Autodesk Inventor part; units mm, degrees
(part 12 of 13)
  line L4314 (13.4922, 7.2115) -> (13.6786, 7.3979)
  arc A4310 (13.6786, 7.3979) -> (13.5708, 7.5057) centre (13.6247, 7.4518) ccw
  line L4315 (13.5708, 7.5057) -> (13.3844, 7.3193)
  arc A4311 (13.3844, 7.3193) -> (13.4922, 7.2115) centre (13.4383, 7.2654) ccw
  line L4316 (13.7009, 7.4518) -> (13.7009, 7.8246)
  arc A4312 (13.7009, 7.8246) -> (13.5485, 7.8246) centre (13.6247, 7.8246) ccw
  line L4317 (13.5485, 7.8246) -> (13.5485, 7.4518)
  arc A4313 (13.5485, 7.4518) -> (13.7009, 7.4518) centre (13.6247, 7.4518) ccw
  line L4318 (13.6786, 7.8785) -> (13.4922, 8.065)
  arc A4314 (13.4922, 8.065) -> (13.3844, 7.9572) centre (13.4383, 8.0111) ccw
  line L4319 (13.3844, 7.9572) -> (13.5708, 7.7707)
  arc A4315 (13.5708, 7.7707) -> (13.6786, 7.8785) centre (13.6247, 7.8246) ccw
  line L4320 (13.4383, 8.0873) -> (12.6926, 8.0873)
  arc A4316 (12.6926, 8.0873) -> (12.6926, 7.9349) centre (12.6926, 8.0111) ccw
  line L4321 (12.6926, 7.9349) -> (13.4383, 7.9349)
  line L4322 (12.6387, 8.065) -> (12.4523, 7.8785)
  arc A4317 (12.4523, 7.8785) -> (12.5601, 7.7707) centre (12.5062, 7.8246) ccw
  line L4323 (12.5601, 7.7707) -> (12.7465, 7.9572)
  arc A4318 (12.7465, 7.9572) -> (12.6387, 8.065) centre (12.6926, 8.0111) ccw
  line L4324 (12.43, 7.8246) -> (12.43, 7.4518)
  arc A4319 (12.43, 7.4518) -> (12.5824, 7.4518) centre (12.5062, 7.4518) ccw
  line L4325 (12.5824, 7.4518) -> (12.5824, 7.8246)
  arc A4320 (12.5824, 7.8246) -> (12.43, 7.8246) centre (12.5062, 7.8246) ccw
  line L4326 (12.4523, 7.3979) -> (12.6387, 7.2115)
  arc A4321 (12.6387, 7.2115) -> (12.7465, 7.3193) centre (12.6926, 7.2654) ccw
  line L4327 (12.7465, 7.3193) -> (12.5601, 7.5057)
  arc A4322 (12.5601, 7.5057) -> (12.4523, 7.3979) centre (12.5062, 7.4518) ccw
  line L4328 (12.7465, 7.2115) -> (13.4922, 7.9572)
  arc A4323 (13.4922, 7.9572) -> (13.3844, 8.065) centre (13.4383, 8.0111) ccw
  line L4329 (13.3844, 8.065) -> (12.6387, 7.3193)
  arc A4324 (12.6387, 7.3193) -> (12.7465, 7.2115) centre (12.6926, 7.2654) ccw
  line L4330 (13.3058, 8.3808) -> (13.6786, 8.7536)
  arc A4325 (13.6786, 8.7536) -> (13.5708, 8.8614) centre (13.6247, 8.8075) ccw
  line L4331 (13.5708, 8.8614) -> (13.198, 8.4886)
  arc A4326 (13.198, 8.4886) -> (13.3058, 8.3808) centre (13.2519, 8.4347) ccw
  line L4332 (13.6247, 8.8837) -> (12.5062, 8.8837)
  arc A4327 (12.5062, 8.8837) -> (12.5062, 8.7313) centre (12.5062, 8.8075) ccw
  line L4333 (12.5062, 8.7313) -> (13.6247, 8.7313)
  arc A4328 (13.6247, 8.7313) -> (13.6247, 8.8837) centre (13.6247, 8.8075) ccw
  line L4334 (12.5824, 8.4347) -> (12.5824, 9.1804)
  arc A4329 (12.5824, 9.1804) -> (12.43, 9.1804) centre (12.5062, 9.1804) ccw
  line L4335 (12.43, 9.1804) -> (12.43, 8.4347)
  arc A4330 (12.43, 8.4347) -> (12.5824, 8.4347) centre (12.5062, 8.4347) ccw
  line L4336 (13.4922, 9.5501) -> (13.6786, 9.7365)
  arc A4331 (13.6786, 9.7365) -> (13.5708, 9.8443) centre (13.6247, 9.7904) ccw
  line L4337 (13.5708, 9.8443) -> (13.3844, 9.6579)
  arc A4332 (13.3844, 9.6579) -> (13.4922, 9.5501) centre (13.4383, 9.604) ccw
  line L4338 (13.7009, 9.7904) -> (13.7009, 10.1632)
  arc A4333 (13.7009, 10.1632) -> (13.5485, 10.1632) centre (13.6247, 10.1632) ccw
  line L4339 (13.5485, 10.1632) -> (13.5485, 9.7904)
  arc A4334 (13.5485, 9.7904) -> (13.7009, 9.7904) centre (13.6247, 9.7904) ccw
  line L4340 (13.6786, 10.2171) -> (13.4922, 10.4036)
  arc A4335 (13.4922, 10.4036) -> (13.3844, 10.2958) centre (13.4383, 10.3497) ccw
  line L4341 (13.3844, 10.2958) -> (13.5708, 10.1093)
  arc A4336 (13.5708, 10.1093) -> (13.6786, 10.2171) centre (13.6247, 10.1632) ccw
  line L4342 (13.4383, 10.4259) -> (13.2519, 10.4259)
  arc A4337 (13.2519, 10.4259) -> (13.2519, 10.2735) centre (13.2519, 10.3497) ccw
  line L4343 (13.2519, 10.2735) -> (13.4383, 10.2735)
  arc A4338 (13.4383, 10.2735) -> (13.4383, 10.4259) centre (13.4383, 10.3497) ccw
  line L4344 (13.198, 10.4036) -> (13.0115, 10.2171)
  arc A4339 (13.0115, 10.2171) -> (13.1193, 10.1093) centre (13.0654, 10.1632) ccw
  line L4345 (13.1193, 10.1093) -> (13.3058, 10.2958)
  arc A4340 (13.3058, 10.2958) -> (13.198, 10.4036) centre (13.2519, 10.3497) ccw
  line L4346 (13.1193, 10.2171) -> (12.9329, 10.4036)
  arc A4341 (12.9329, 10.4036) -> (12.8251, 10.2958) centre (12.879, 10.3497) ccw
  line L4347 (12.8251, 10.2958) -> (13.0115, 10.1093)
  arc A4342 (13.0115, 10.1093) -> (13.1193, 10.2171) centre (13.0654, 10.1632) ccw
  line L4348 (12.879, 10.4259) -> (12.6926, 10.4259)
  arc A4343 (12.6926, 10.4259) -> (12.6926, 10.2735) centre (12.6926, 10.3497) ccw
  line L4349 (12.6926, 10.2735) -> (12.879, 10.2735)
  arc A4344 (12.879, 10.2735) -> (12.879, 10.4259) centre (12.879, 10.3497) ccw
  line L4350 (12.6387, 10.4036) -> (12.4523, 10.2171)
  arc A4345 (12.4523, 10.2171) -> (12.5601, 10.1093) centre (12.5062, 10.1632) ccw
  line L4351 (12.5601, 10.1093) -> (12.7465, 10.2958)
  arc A4346 (12.7465, 10.2958) -> (12.6387, 10.4036) centre (12.6926, 10.3497) ccw
  line L4352 (12.43, 10.1632) -> (12.43, 9.7904)
  arc A4347 (12.43, 9.7904) -> (12.5824, 9.7904) centre (12.5062, 9.7904) ccw
  line L4353 (12.5824, 9.7904) -> (12.5824, 10.1632)
  arc A4348 (12.5824, 10.1632) -> (12.43, 10.1632) centre (12.5062, 10.1632) ccw
  line L4354 (12.4523, 9.7365) -> (12.6387, 9.5501)
  arc A4349 (12.6387, 9.5501) -> (12.7465, 9.6579) centre (12.6926, 9.604) ccw
  line L4355 (12.7465, 9.6579) -> (12.5601, 9.8443)
  arc A4350 (12.5601, 9.8443) -> (12.4523, 9.7365) centre (12.5062, 9.7904) ccw
  line L4356 (12.6926, 9.5278) -> (12.879, 9.5278)
  arc A4351 (12.879, 9.5278) -> (12.879, 9.6802) centre (12.879, 9.604) ccw
  line L4357 (12.879, 9.6802) -> (12.6926, 9.6802)
  arc A4352 (12.6926, 9.6802) -> (12.6926, 9.5278) centre (12.6926, 9.604) ccw
  line L4358 (12.9329, 9.5501) -> (13.1193, 9.7365)
  arc A4353 (13.1193, 9.7365) -> (13.0115, 9.8443) centre (13.0654, 9.7904) ccw
  line L4359 (13.0115, 9.8443) -> (12.8251, 9.6579)
  arc A4354 (12.8251, 9.6579) -> (12.9329, 9.5501) centre (12.879, 9.604) ccw
  line L4360 (13.0115, 9.7365) -> (13.198, 9.5501)
  arc A4355 (13.198, 9.5501) -> (13.3058, 9.6579) centre (13.2519, 9.604) ccw
  line L4361 (13.3058, 9.6579) -> (13.1193, 9.8443)
  arc A4356 (13.1193, 9.8443) -> (13.0115, 9.7365) centre (13.0654, 9.7904) ccw
  line L4362 (13.2519, 9.5278) -> (13.4383, 9.5278)
  arc A4357 (13.4383, 9.5278) -> (13.4383, 9.6802) centre (13.4383, 9.604) ccw
  line L4363 (13.4383, 9.6802) -> (13.2519, 9.6802)
  arc A4358 (13.2519, 9.6802) -> (13.2519, 9.5278) centre (13.2519, 9.604) ccw
  line L4364 (13.1416, 9.7904) -> (13.1416, 10.1632)
  arc A4359 (13.1416, 10.1632) -> (12.9892, 10.1632) centre (13.0654, 10.1632) ccw
  line L4365 (12.9892, 10.1632) -> (12.9892, 9.7904)
  arc A4360 (12.9892, 9.7904) -> (13.1416, 9.7904) centre (13.0654, 9.7904) ccw
  line L4366 (12.5062, 11.8664) -> (13.6247, 11.8664)
  arc A4361 (13.6247, 11.8664) -> (13.6247, 12.0188) centre (13.6247, 11.9426) ccw
  line L4367 (13.6247, 12.0188) -> (12.5062, 12.0188)
  arc A4362 (12.5062, 12.0188) -> (12.5062, 11.8664) centre (12.5062, 11.9426) ccw
  line L4368 (13.7009, 11.9426) -> (13.7009, 12.5018)
  arc A4363 (13.7009, 12.5018) -> (13.5485, 12.5018) centre (13.6247, 12.5018) ccw
  line L4369 (13.5485, 12.5018) -> (13.5485, 11.9426)
  arc A4364 (13.5485, 11.9426) -> (13.7009, 11.9426) centre (13.6247, 11.9426) ccw
  line L4370 (13.6786, 12.5557) -> (13.4922, 12.7422)
  arc A4365 (13.4922, 12.7422) -> (13.3844, 12.6344) centre (13.4383, 12.6883) ccw
  line L4371 (13.3844, 12.6344) -> (13.5708, 12.4479)
  arc A4366 (13.5708, 12.4479) -> (13.6786, 12.5557) centre (13.6247, 12.5018) ccw
  line L4372 (13.4383, 12.7645) -> (13.0654, 12.7645)
  arc A4367 (13.0654, 12.7645) -> (13.0654, 12.6121) centre (13.0654, 12.6883) ccw
  line L4373 (13.0654, 12.6121) -> (13.4383, 12.6121)
  arc A4368 (13.4383, 12.6121) -> (13.4383, 12.7645) centre (13.4383, 12.6883) ccw
  line L4374 (13.0115, 12.7422) -> (12.8251, 12.5557)
  arc A4369 (12.8251, 12.5557) -> (12.9329, 12.4479) centre (12.879, 12.5018) ccw
  line L4375 (12.9329, 12.4479) -> (13.1193, 12.6344)
  arc A4370 (13.1193, 12.6344) -> (13.0115, 12.7422) centre (13.0654, 12.6883) ccw
  line L4376 (12.8028, 12.5018) -> (12.8028, 11.9426)
  arc A4371 (12.8028, 11.9426) -> (12.9552, 11.9426) centre (12.879, 11.9426) ccw
  line L4377 (12.9552, 11.9426) -> (12.9552, 12.5018)
  arc A4372 (12.9552, 12.5018) -> (12.8028, 12.5018) centre (12.879, 12.5018) ccw
  line L4378 (12.9329, 12.3693) -> (12.5601, 12.7422)
  arc A4373 (12.5601, 12.7422) -> (12.4523, 12.6344) centre (12.5062, 12.6883) ccw
  line L4379 (12.4523, 12.6344) -> (12.8251, 12.2615)
  arc A4374 (12.8251, 12.2615) -> (12.9329, 12.3693) centre (12.879, 12.3154) ccw
  line L4380 (12.5062, 14.205) -> (13.6247, 14.205)
  arc A4375 (13.6247, 14.205) -> (13.6247, 14.3574) centre (13.6247, 14.2812) ccw
  line L4381 (13.6247, 14.3574) -> (12.5062, 14.3574)
  arc A4376 (12.5062, 14.3574) -> (12.5062, 14.205) centre (12.5062, 14.2812) ccw
  line L4382 (13.7009, 14.2812) -> (13.7009, 14.8404)
  arc A4377 (13.7009, 14.8404) -> (13.5485, 14.8404) centre (13.6247, 14.8404) ccw
  line L4383 (13.5485, 14.8404) -> (13.5485, 14.2812)
  arc A4378 (13.5485, 14.2812) -> (13.7009, 14.2812) centre (13.6247, 14.2812) ccw
  line L4384 (13.6786, 14.8943) -> (13.4922, 15.0808)
  arc A4379 (13.4922, 15.0808) -> (13.3844, 14.973) centre (13.4383, 15.0269) ccw
  line L4385 (13.3844, 14.973) -> (13.5708, 14.7865)
  arc A4380 (13.5708, 14.7865) -> (13.6786, 14.8943) centre (13.6247, 14.8404) ccw
  line L4386 (13.4383, 15.1031) -> (13.0654, 15.1031)
  arc A4381 (13.0654, 15.1031) -> (13.0654, 14.9507) centre (13.0654, 15.0269) ccw
  line L4387 (13.0654, 14.9507) -> (13.4383, 14.9507)
  arc A4382 (13.4383, 14.9507) -> (13.4383, 15.1031) centre (13.4383, 15.0269) ccw
  line L4388 (13.0115, 15.0808) -> (12.8251, 14.8943)
  arc A4383 (12.8251, 14.8943) -> (12.9329, 14.7865) centre (12.879, 14.8404) ccw
  line L4389 (12.9329, 14.7865) -> (13.1193, 14.973)
  arc A4384 (13.1193, 14.973) -> (13.0115, 15.0808) centre (13.0654, 15.0269) ccw
  line L4390 (12.8028, 14.8404) -> (12.8028, 14.2812)
  arc A4385 (12.8028, 14.2812) -> (12.9552, 14.2812) centre (12.879, 14.2812) ccw
  line L4391 (12.9552, 14.2812) -> (12.9552, 14.8404)
  arc A4386 (12.9552, 14.8404) -> (12.8028, 14.8404) centre (12.879, 14.8404) ccw
  line L4392 (12.9329, 14.7079) -> (12.5601, 15.0808)
  arc A4387 (12.5601, 15.0808) -> (12.4523, 14.973) centre (12.5062, 15.0269) ccw
  line L4393 (12.4523, 14.973) -> (12.8251, 14.6001)
  arc A4388 (12.8251, 14.6001) -> (12.9329, 14.7079) centre (12.879, 14.654) ccw
  line L4394 (12.5062, 15.3743) -> (13.2519, 15.3743)
  arc A4389 (13.2519, 15.3743) -> (13.2519, 15.5267) centre (13.2519, 15.4505) ccw
  line L4395 (13.2519, 15.5267) -> (12.5062, 15.5267)
  arc A4390 (12.5062, 15.5267) -> (12.5062, 15.3743) centre (12.5062, 15.4505) ccw
  line L4396 (13.3058, 15.3966) -> (13.6786, 15.7694)
  arc A4391 (13.6786, 15.7694) -> (13.5708, 15.8772) centre (13.6247, 15.8233) ccw
  line L4397 (13.5708, 15.8772) -> (13.198, 15.5044)
  arc A4392 (13.198, 15.5044) -> (13.3058, 15.3966) centre (13.2519, 15.4505) ccw
  line L4398 (13.6786, 15.8772) -> (13.3058, 16.2501)
  arc A4393 (13.3058, 16.2501) -> (13.198, 16.1423) centre (13.2519, 16.1962) ccw
  line L4399 (13.198, 16.1423) -> (13.5708, 15.7694)
  arc A4394 (13.5708, 15.7694) -> (13.6786, 15.8772) centre (13.6247, 15.8233) ccw
  line L4400 (13.2519, 16.2724) -> (12.5062, 16.2724)
  arc A4395 (12.5062, 16.2724) -> (12.5062, 16.12) centre (12.5062, 16.1962) ccw
  line L4401 (12.5062, 16.12) -> (13.2519, 16.12)
  arc A4396 (13.2519, 16.12) -> (13.2519, 16.2724) centre (13.2519, 16.1962) ccw
  line L4402 (13.1416, 15.4505) -> (13.1416, 16.1962)
  arc A4397 (13.1416, 16.1962) -> (12.9892, 16.1962) centre (13.0654, 16.1962) ccw
  line L4403 (12.9892, 16.1962) -> (12.9892, 15.4505)
  arc A4398 (12.9892, 15.4505) -> (13.1416, 15.4505) centre (13.0654, 15.4505) ccw
  line L4404 (13.6247, 16.696) -> (12.5062, 16.696)
  arc A4399 (12.5062, 16.696) -> (12.5062, 16.5436) centre (12.5062, 16.6198) ccw
  line L4405 (12.5062, 16.5436) -> (13.6247, 16.5436)
  arc A4400 (13.6247, 16.5436) -> (13.6247, 16.696) centre (13.6247, 16.6198) ccw
  line L4406 (12.5824, 16.6198) -> (12.5824, 17.179)
  arc A4401 (12.5824, 17.179) -> (12.43, 17.179) centre (12.5062, 17.179) ccw
  line L4407 (12.43, 17.179) -> (12.43, 16.6198)
  arc A4402 (12.43, 16.6198) -> (12.5824, 16.6198) centre (12.5062, 16.6198) ccw
  line L4408 (12.5601, 17.1251) -> (12.7465, 17.3116)
  arc A4403 (12.7465, 17.3116) -> (12.6387, 17.4194) centre (12.6926, 17.3655) ccw
  line L4409 (12.6387, 17.4194) -> (12.4523, 17.2329)
  arc A4404 (12.4523, 17.2329) -> (12.5601, 17.1251) centre (12.5062, 17.179) ccw
  line L4410 (12.6926, 17.2893) -> (13.4383, 17.2893)
  arc A4405 (13.4383, 17.2893) -> (13.4383, 17.4417) centre (13.4383, 17.3655) ccw
  line L4411 (13.4383, 17.4417) -> (12.6926, 17.4417)
  arc A4406 (12.6926, 17.4417) -> (12.6926, 17.2893) centre (12.6926, 17.3655) ccw
  line L4412 (13.3844, 17.3116) -> (13.5708, 17.1251)
  arc A4407 (13.5708, 17.1251) -> (13.6786, 17.2329) centre (13.6247, 17.179) ccw
  line L4413 (13.6786, 17.2329) -> (13.4922, 17.4194)
  arc A4408 (13.4922, 17.4194) -> (13.3844, 17.3116) centre (13.4383, 17.3655) ccw
  line L4414 (13.5485, 17.179) -> (13.5485, 16.6198)
  arc A4409 (13.5485, 16.6198) -> (13.7009, 16.6198) centre (13.6247, 16.6198) ccw
  line L4415 (13.7009, 16.6198) -> (13.7009, 17.179)
  arc A4410 (13.7009, 17.179) -> (13.5485, 17.179) centre (13.6247, 17.179) ccw
  line L4416 (13.5485, 18.5348) -> (13.5485, 17.7891)
  arc A4411 (13.5485, 17.7891) -> (13.7009, 17.7891) centre (13.6247, 17.7891) ccw
  line L4417 (13.7009, 17.7891) -> (13.7009, 18.5348)
  arc A4412 (13.7009, 18.5348) -> (13.5485, 18.5348) centre (13.6247, 18.5348) ccw
  line L4418 (13.6247, 17.8653) -> (12.5062, 17.8653)
  arc A4413 (12.5062, 17.8653) -> (12.5062, 17.7129) centre (12.5062, 17.7891) ccw
  line L4419 (12.5062, 17.7129) -> (13.6247, 17.7129)
  arc A4414 (13.6247, 17.7129) -> (13.6247, 17.8653) centre (13.6247, 17.7891) ccw
  line L4420 (12.5824, 17.7891) -> (12.5824, 18.5348)
  arc A4415 (12.5824, 18.5348) -> (12.43, 18.5348) centre (12.5062, 18.5348) ccw
  line L4421 (12.43, 18.5348) -> (12.43, 17.7891)
  arc A4416 (12.43, 17.7891) -> (12.5824, 17.7891) centre (12.5062, 17.7891) ccw
  line L4422 (13.1416, 17.7891) -> (13.1416, 18.1619)
  arc A4417 (13.1416, 18.1619) -> (12.9892, 18.1619) centre (13.0654, 18.1619) ccw
  line L4423 (12.9892, 18.1619) -> (12.9892, 17.7891)
  arc A4418 (12.9892, 17.7891) -> (13.1416, 17.7891) centre (13.0654, 17.7891) ccw
  line L4424 (12.5062, 18.8822) -> (13.6247, 18.8822)
  arc A4419 (13.6247, 18.8822) -> (13.6247, 19.0346) centre (13.6247, 18.9584) ccw
  line L4425 (13.6247, 19.0346) -> (12.5062, 19.0346)
  arc A4420 (12.5062, 19.0346) -> (12.5062, 18.8822) centre (12.5062, 18.9584) ccw
  line L4426 (13.6786, 19.0123) -> (13.3058, 19.3851)
  arc A4421 (13.3058, 19.3851) -> (13.198, 19.2773) centre (13.2519, 19.3312) ccw
  line L4427 (13.198, 19.2773) -> (13.5708, 18.9045)
  arc A4422 (13.5708, 18.9045) -> (13.6786, 19.0123) centre (13.6247, 18.9584) ccw
  line L4428 (13.3058, 19.2773) -> (13.6786, 19.6502)
  arc A4423 (13.6786, 19.6502) -> (13.5708, 19.758) centre (13.6247, 19.7041) ccw
  line L4429 (13.5708, 19.758) -> (13.198, 19.3851)
  arc A4424 (13.198, 19.3851) -> (13.3058, 19.2773) centre (13.2519, 19.3312) ccw
  line L4430 (13.6247, 19.7803) -> (12.5062, 19.7803)
  arc A4425 (12.5062, 19.7803) -> (12.5062, 19.6279) centre (12.5062, 19.7041) ccw
  line L4431 (12.5062, 19.6279) -> (13.6247, 19.6279)
  arc A4426 (13.6247, 19.6279) -> (13.6247, 19.7803) centre (13.6247, 19.7041) ccw
  line L4432 (12.5062, 20.0515) -> (13.2519, 20.0515)
  arc A4427 (13.2519, 20.0515) -> (13.2519, 20.2039) centre (13.2519, 20.1277) ccw
  line L4433 (13.2519, 20.2039) -> (12.5062, 20.2039)
  arc A4428 (12.5062, 20.2039) -> (12.5062, 20.0515) centre (12.5062, 20.1277) ccw
  line L4434 (13.3058, 20.0738) -> (13.6786, 20.4466)
  arc A4429 (13.6786, 20.4466) -> (13.5708, 20.5544) centre (13.6247, 20.5005) ccw
  line L4435 (13.5708, 20.5544) -> (13.198, 20.1816)
  arc A4430 (13.198, 20.1816) -> (13.3058, 20.0738) centre (13.2519, 20.1277) ccw
  line L4436 (13.6786, 20.5544) -> (13.3058, 20.9273)
  arc A4431 (13.3058, 20.9273) -> (13.198, 20.8195) centre (13.2519, 20.8734) ccw
  line L4437 (13.198, 20.8195) -> (13.5708, 20.4466)
  arc A4432 (13.5708, 20.4466) -> (13.6786, 20.5544) centre (13.6247, 20.5005) ccw
  line L4438 (13.2519, 20.9496) -> (12.5062, 20.9496)
  arc A4433 (12.5062, 20.9496) -> (12.5062, 20.7972) centre (12.5062, 20.8734) ccw
  line L4439 (12.5062, 20.7972) -> (13.2519, 20.7972)
  arc A4434 (13.2519, 20.7972) -> (13.2519, 20.9496) centre (13.2519, 20.8734) ccw
  line L4440 (13.1416, 20.1277) -> (13.1416, 20.8734)
  arc A4435 (13.1416, 20.8734) -> (12.9892, 20.8734) centre (13.0654, 20.8734) ccw
  line L4441 (12.9892, 20.8734) -> (12.9892, 20.1277)
  arc A4436 (12.9892, 20.1277) -> (13.1416, 20.1277) centre (13.0654, 20.1277) ccw
  line L4442 (13.3844, 21.9888) -> (13.5708, 21.8023)
  arc A4437 (13.5708, 21.8023) -> (13.6786, 21.9101) centre (13.6247, 21.8562) ccw
  line L4443 (13.6786, 21.9101) -> (13.4922, 22.0966)
  arc A4438 (13.4922, 22.0966) -> (13.3844, 21.9888) centre (13.4383, 22.0427) ccw
  line L4444 (13.5485, 21.8562) -> (13.5485, 21.4834)
  arc A4439 (13.5485, 21.4834) -> (13.7009, 21.4834) centre (13.6247, 21.4834) ccw
  line L4445 (13.7009, 21.4834) -> (13.7009, 21.8562)
  arc A4440 (13.7009, 21.8562) -> (13.5485, 21.8562) centre (13.6247, 21.8562) ccw
  line L4446 (13.5708, 21.5373) -> (13.3844, 21.3509)
  arc A4441 (13.3844, 21.3509) -> (13.4922, 21.2431) centre (13.4383, 21.297) ccw
  line L4447 (13.4922, 21.2431) -> (13.6786, 21.4295)
  arc A4442 (13.6786, 21.4295) -> (13.5708, 21.5373) centre (13.6247, 21.4834) ccw
  line L4448 (13.4383, 21.3732) -> (12.6926, 21.3732)
  arc A4443 (12.6926, 21.3732) -> (12.6926, 21.2208) centre (12.6926, 21.297) ccw
  line L4449 (12.6926, 21.2208) -> (13.4383, 21.2208)
  arc A4444 (13.4383, 21.2208) -> (13.4383, 21.3732) centre (13.4383, 21.297) ccw
  line L4450 (12.7465, 21.3509) -> (12.5601, 21.5373)
  arc A4445 (12.5601, 21.5373) -> (12.4523, 21.4295) centre (12.5062, 21.4834) ccw
  line L4451 (12.4523, 21.4295) -> (12.6387, 21.2431)
  arc A4446 (12.6387, 21.2431) -> (12.7465, 21.3509) centre (12.6926, 21.297) ccw
  line L4452 (12.5824, 21.4834) -> (12.5824, 21.8562)
  arc A4447 (12.5824, 21.8562) -> (12.43, 21.8562) centre (12.5062, 21.8562) ccw
  line L4453 (12.43, 21.8562) -> (12.43, 21.4834)
  arc A4448 (12.43, 21.4834) -> (12.5824, 21.4834) centre (12.5062, 21.4834) ccw
  line L4454 (12.5601, 21.8023) -> (12.7465, 21.9888)
  arc A4449 (12.7465, 21.9888) -> (12.6387, 22.0966) centre (12.6926, 22.0427) ccw
  line L4455 (12.6387, 22.0966) -> (12.4523, 21.9101)
  arc A4450 (12.4523, 21.9101) -> (12.5601, 21.8023) centre (12.5062, 21.8562) ccw
  line L4456 (12.5062, 22.3901) -> (13.6247, 22.3901)
  arc A4451 (13.6247, 22.3901) -> (13.6247, 22.5425) centre (13.6247, 22.4663) ccw
  line L4457 (13.6247, 22.5425) -> (12.5062, 22.5425)
  arc A4452 (12.5062, 22.5425) -> (12.5062, 22.3901) centre (12.5062, 22.4663) ccw
  line L4458 (13.1416, 22.4663) -> (13.1416, 23.212)
  arc A4453 (13.1416, 23.212) -> (12.9892, 23.212) centre (13.0654, 23.212) ccw
  line L4459 (12.9892, 23.212) -> (12.9892, 22.4663)
  arc A4454 (12.9892, 22.4663) -> (13.1416, 22.4663) centre (13.0654, 22.4663) ccw
  line L4460 (13.6247, 23.2882) -> (12.5062, 23.2882)
  arc A4455 (12.5062, 23.2882) -> (12.5062, 23.1358) centre (12.5062, 23.212) ccw
  line L4461 (12.5062, 23.1358) -> (13.6247, 23.1358)
  arc A4456 (13.6247, 23.1358) -> (13.6247, 23.2882) centre (13.6247, 23.212) ccw
  line L4462 (13.5485, 24.3813) -> (13.5485, 23.6356)
  arc A4457 (13.5485, 23.6356) -> (13.7009, 23.6356) centre (13.6247, 23.6356) ccw
  line L4463 (13.7009, 23.6356) -> (13.7009, 24.3813)
  arc A4458 (13.7009, 24.3813) -> (13.5485, 24.3813) centre (13.6247, 24.3813) ccw
  line L4464 (13.6247, 23.7118) -> (12.5062, 23.7118)
  arc A4459 (12.5062, 23.7118) -> (12.5062, 23.5594) centre (12.5062, 23.6356) ccw
  line L4465 (12.5062, 23.5594) -> (13.6247, 23.5594)
  arc A4460 (13.6247, 23.5594) -> (13.6247, 23.7118) centre (13.6247, 23.6356) ccw
  line L4466 (12.5824, 23.6356) -> (12.5824, 24.3813)
  arc A4461 (12.5824, 24.3813) -> (12.43, 24.3813) centre (12.5062, 24.3813) ccw
  line L4467 (12.43, 24.3813) -> (12.43, 23.6356)
  arc A4462 (12.43, 23.6356) -> (12.5824, 23.6356) centre (12.5062, 23.6356) ccw
  line L4468 (13.1416, 23.6356) -> (13.1416, 24.0084)
  arc A4463 (13.1416, 24.0084) -> (12.9892, 24.0084) centre (13.0654, 24.0084) ccw
  line L4469 (12.9892, 24.0084) -> (12.9892, 23.6356)
  arc A4464 (12.9892, 23.6356) -> (13.1416, 23.6356) centre (13.0654, 23.6356) ccw
  line L4470 (12.5062, 24.7287) -> (13.6247, 24.7287)
  arc A4465 (13.6247, 24.7287) -> (13.6247, 24.8811) centre (13.6247, 24.8049) ccw
  line L4471 (13.6247, 24.8811) -> (12.5062, 24.8811)
  arc A4466 (12.5062, 24.8811) -> (12.5062, 24.7287) centre (12.5062, 24.8049) ccw
  line L4472 (13.7009, 24.8049) -> (13.7009, 25.3641)
  arc A4467 (13.7009, 25.3641) -> (13.5485, 25.3641) centre (13.6247, 25.3641) ccw
  line L4473 (13.5485, 25.3641) -> (13.5485, 24.8049)
  arc A4468 (13.5485, 24.8049) -> (13.7009, 24.8049) centre (13.6247, 24.8049) ccw
  line L4474 (13.6786, 25.418) -> (13.4922, 25.6045)
  arc A4469 (13.4922, 25.6045) -> (13.3844, 25.4967) centre (13.4383, 25.5506) ccw
  line L4475 (13.3844, 25.4967) -> (13.5708, 25.3102)
  arc A4470 (13.5708, 25.3102) -> (13.6786, 25.418) centre (13.6247, 25.3641) ccw
  line L4476 (13.4383, 25.6268) -> (13.0654, 25.6268)
  arc A4471 (13.0654, 25.6268) -> (13.0654, 25.4744) centre (13.0654, 25.5506) ccw
  line L4477 (13.0654, 25.4744) -> (13.4383, 25.4744)
  arc A4472 (13.4383, 25.4744) -> (13.4383, 25.6268) centre (13.4383, 25.5506) ccw
  line L4478 (13.0115, 25.6045) -> (12.8251, 25.418)
  arc A4473 (12.8251, 25.418) -> (12.9329, 25.3102) centre (12.879, 25.3641) ccw
  line L4479 (12.9329, 25.3102) -> (13.1193, 25.4967)
  arc A4474 (13.1193, 25.4967) -> (13.0115, 25.6045) centre (13.0654, 25.5506) ccw
  line L4480 (12.8028, 25.3641) -> (12.8028, 24.8049)
  arc A4475 (12.8028, 24.8049) -> (12.9552, 24.8049) centre (12.879, 24.8049) ccw
  line L4481 (12.9552, 24.8049) -> (12.9552, 25.3641)
  arc A4476 (12.9552, 25.3641) -> (12.8028, 25.3641) centre (12.879, 25.3641) ccw
  line L4482 (12.9329, 25.2316) -> (12.5601, 25.6045)
  arc A4477 (12.5601, 25.6045) -> (12.4523, 25.4967) centre (12.5062, 25.5506) ccw
  line L4483 (12.4523, 25.4967) -> (12.8251, 25.1238)
  arc A4478 (12.8251, 25.1238) -> (12.9329, 25.2316) centre (12.879, 25.1777) ccw
  line L4484 (13.6947, 29.1524) -> (12.7626, 29.1524)
  arc A4479 (12.7626, 29.1524) -> (12.7626, 29) centre (12.7626, 29.0762) ccw
  line L4485 (12.7626, 29) -> (13.6947, 29)
  arc A4480 (13.6947, 29) -> (13.6947, 29.1524) centre (13.6947, 29.0762) ccw
  line L4486 (12.8165, 29.1301) -> (12.6301, 29.3165)
  arc A4481 (12.6301, 29.3165) -> (12.5223, 29.2087) centre (12.5762, 29.2626) ccw
  line L4487 (12.5223, 29.2087) -> (12.7087, 29.0223)
  arc A4482 (12.7087, 29.0223) -> (12.8165, 29.1301) centre (12.7626, 29.0762) ccw
  line L4488 (12.6524, 29.2626) -> (12.6524, 29.6354)
  arc A4483 (12.6524, 29.6354) -> (12.5, 29.6354) centre (12.5762, 29.6354) ccw
  line L4489 (12.5, 29.6354) -> (12.5, 29.2626)
  arc A4484 (12.5, 29.2626) -> (12.6524, 29.2626) centre (12.5762, 29.2626) ccw
  line L4490 (12.6301, 29.5815) -> (12.8165, 29.768)
  arc A4485 (12.8165, 29.768) -> (12.7087, 29.8758) centre (12.7626, 29.8219) ccw
  line L4491 (12.7087, 29.8758) -> (12.5223, 29.6893)
  arc A4486 (12.5223, 29.6893) -> (12.6301, 29.5815) centre (12.5762, 29.6354) ccw
  line L4492 (12.7626, 29.7457) -> (13.6947, 29.7457)
  arc A4487 (13.6947, 29.7457) -> (13.6947, 29.8981) centre (13.6947, 29.8219) ccw
  line L4493 (13.6947, 29.8981) -> (12.7626, 29.8981)
  arc A4488 (12.7626, 29.8981) -> (12.7626, 29.7457) centre (12.7626, 29.8219) ccw
  line L4494 (13.6947, 30.3217) -> (12.5762, 30.3217)
  arc A4489 (12.5762, 30.3217) -> (12.5762, 30.1693) centre (12.5762, 30.2455) ccw
  line L4495 (12.5762, 30.1693) -> (13.6947, 30.1693)
  arc A4490 (13.6947, 30.1693) -> (13.6947, 30.3217) centre (13.6947, 30.2455) ccw
  line L4496 (12.6301, 30.1916) -> (13.0029, 30.5644)
  arc A4491 (13.0029, 30.5644) -> (12.8951, 30.6722) centre (12.949, 30.6183) ccw
  line L4497 (12.8951, 30.6722) -> (12.5223, 30.2994)
  arc A4492 (12.5223, 30.2994) -> (12.6301, 30.1916) centre (12.5762, 30.2455) ccw
  line L4498 (13.0029, 30.6722) -> (12.6301, 31.0451)
  arc A4493 (12.6301, 31.0451) -> (12.5223, 30.9373) centre (12.5762, 30.9912) ccw
  line L4499 (12.5223, 30.9373) -> (12.8951, 30.5644)
  arc A4494 (12.8951, 30.5644) -> (13.0029, 30.6722) centre (12.949, 30.6183) ccw
  line L4500 (12.5762, 30.915) -> (13.6947, 30.915)
  arc A4495 (13.6947, 30.915) -> (13.6947, 31.0674) centre (13.6947, 30.9912) ccw
  line L4501 (13.6947, 31.0674) -> (12.5762, 31.0674)
  arc A4496 (12.5762, 31.0674) -> (12.5762, 30.915) centre (12.5762, 30.9912) ccw
  line L4502 (12.5762, 31.3386) -> (13.3219, 31.3386)
  arc A4497 (13.3219, 31.3386) -> (13.3219, 31.491) centre (13.3219, 31.4148) ccw
  line L4503 (13.3219, 31.491) -> (12.5762, 31.491)
  arc A4498 (12.5762, 31.491) -> (12.5762, 31.3386) centre (12.5762, 31.4148) ccw
  line L4504 (13.3758, 31.3609) -> (13.7486, 31.7337)
  arc A4499 (13.7486, 31.7337) -> (13.6408, 31.8415) centre (13.6947, 31.7876) ccw
  line L4505 (13.6408, 31.8415) -> (13.268, 31.4687)
  arc A4500 (13.268, 31.4687) -> (13.3758, 31.3609) centre (13.3219, 31.4148) ccw
  line L4506 (13.7486, 31.8415) -> (13.3758, 32.2144)
  arc A4501 (13.3758, 32.2144) -> (13.268, 32.1066) centre (13.3219, 32.1605) ccw
  line L4507 (13.268, 32.1066) -> (13.6408, 31.7337)
  arc A4502 (13.6408, 31.7337) -> (13.7486, 31.8415) centre (13.6947, 31.7876) ccw
  line L4508 (13.3219, 32.2367) -> (12.5762, 32.2367)
  arc A4503 (12.5762, 32.2367) -> (12.5762, 32.0843) centre (12.5762, 32.1605) ccw
  line L4509 (12.5762, 32.0843) -> (13.3219, 32.0843)
  arc A4504 (13.3219, 32.0843) -> (13.3219, 32.2367) centre (13.3219, 32.1605) ccw
  line L4510 (13.2116, 31.4148) -> (13.2116, 32.1605)
  arc A4505 (13.2116, 32.1605) -> (13.0592, 32.1605) centre (13.1354, 32.1605) ccw
  line L4511 (13.0592, 32.1605) -> (13.0592, 31.4148)
  arc A4506 (13.0592, 31.4148) -> (13.2116, 31.4148) centre (13.1354, 31.4148) ccw
  line L4512 (12.5762, 32.8807) -> (13.6947, 32.8807)
  arc A4507 (13.6947, 32.8807) -> (13.6947, 33.0331) centre (13.6947, 32.9569) ccw
  line L4513 (13.6947, 33.0331) -> (12.5762, 33.0331)
  arc A4508 (12.5762, 33.0331) -> (12.5762, 32.8807) centre (12.5762, 32.9569) ccw
  line L4514 (13.7709, 32.5841) -> (13.7709, 33.3298)
  arc A4509 (13.7709, 33.3298) -> (13.6185, 33.3298) centre (13.6947, 33.3298) ccw
  line L4515 (13.6185, 33.3298) -> (13.6185, 32.5841)
  arc A4510 (13.6185, 32.5841) -> (13.7709, 32.5841) centre (13.6947, 32.5841) ccw
  line L4516 (13.6185, 34.4991) -> (13.6185, 33.7534)
  arc A4511 (13.6185, 33.7534) -> (13.7709, 33.7534) centre (13.6947, 33.7534) ccw
  line L4517 (13.7709, 33.7534) -> (13.7709, 34.4991)
  arc A4512 (13.7709, 34.4991) -> (13.6185, 34.4991) centre (13.6947, 34.4991) ccw
  line L4518 (13.6947, 33.8296) -> (12.5762, 33.8296)
  arc A4513 (12.5762, 33.8296) -> (12.5762, 33.6772) centre (12.5762, 33.7534) ccw
  line L4519 (12.5762, 33.6772) -> (13.6947, 33.6772)
  arc A4514 (13.6947, 33.6772) -> (13.6947, 33.8296) centre (13.6947, 33.7534) ccw
  line L4520 (12.6524, 33.7534) -> (12.6524, 34.4991)
  arc A4515 (12.6524, 34.4991) -> (12.5, 34.4991) centre (12.5762, 34.4991) ccw
  line L4521 (12.5, 34.4991) -> (12.5, 33.7534)
  arc A4516 (12.5, 33.7534) -> (12.6524, 33.7534) centre (12.5762, 33.7534) ccw
  line L4522 (13.2116, 33.7534) -> (13.2116, 34.1262)
  arc A4517 (13.2116, 34.1262) -> (13.0592, 34.1262) centre (13.1354, 34.1262) ccw
  line L4523 (13.0592, 34.1262) -> (13.0592, 33.7534)
  arc A4518 (13.0592, 33.7534) -> (13.2116, 33.7534) centre (13.1354, 33.7534) ccw
  line L4524 (12.5762, 34.8465) -> (13.6947, 34.8465)
  arc A4519 (13.6947, 34.8465) -> (13.6947, 34.9989) centre (13.6947, 34.9227) ccw
  line L4525 (13.6947, 34.9989) -> (12.5762, 34.9989)
  arc A4520 (12.5762, 34.9989) -> (12.5762, 34.8465) centre (12.5762, 34.9227) ccw
  line L4526 (13.7709, 34.9227) -> (13.7709, 35.4819)
  arc A4521 (13.7709, 35.4819) -> (13.6185, 35.4819) centre (13.6947, 35.4819) ccw
  line L4527 (13.6185, 35.4819) -> (13.6185, 34.9227)
  arc A4522 (13.6185, 34.9227) -> (13.7709, 34.9227) centre (13.6947, 34.9227) ccw
  line L4528 (13.7486, 35.5358) -> (13.5622, 35.7223)
  arc A4523 (13.5622, 35.7223) -> (13.4544, 35.6145) centre (13.5083, 35.6684) ccw
  line L4529 (13.4544, 35.6145) -> (13.6408, 35.428)
  arc A4524 (13.6408, 35.428) -> (13.7486, 35.5358) centre (13.6947, 35.4819) ccw
  line L4530 (13.5083, 35.7446) -> (13.1354, 35.7446)
  arc A4525 (13.1354, 35.7446) -> (13.1354, 35.5922) centre (13.1354, 35.6684) ccw
  line L4531 (13.1354, 35.5922) -> (13.5083, 35.5922)
  arc A4526 (13.5083, 35.5922) -> (13.5083, 35.7446) centre (13.5083, 35.6684) ccw
  line L4532 (13.0815, 35.7223) -> (12.8951, 35.5358)
  arc A4527 (12.8951, 35.5358) -> (13.0029, 35.428) centre (12.949, 35.4819) ccw
  line L4533 (13.0029, 35.428) -> (13.1893, 35.6145)
  arc A4528 (13.1893, 35.6145) -> (13.0815, 35.7223) centre (13.1354, 35.6684) ccw
  line L4534 (12.8728, 35.4819) -> (12.8728, 34.9227)
  arc A4529 (12.8728, 34.9227) -> (13.0252, 34.9227) centre (12.949, 34.9227) ccw
  line L4535 (13.0252, 34.9227) -> (13.0252, 35.4819)
  arc A4530 (13.0252, 35.4819) -> (12.8728, 35.4819) centre (12.949, 35.4819) ccw
  line L4536 (13.0029, 35.3494) -> (12.6301, 35.7223)
  arc A4531 (12.6301, 35.7223) -> (12.5223, 35.6145) centre (12.5762, 35.6684) ccw
  line L4537 (12.5223, 35.6145) -> (12.8951, 35.2416)
  arc A4532 (12.8951, 35.2416) -> (13.0029, 35.3494) centre (12.949, 35.2955) ccw
  line L4538 (13.6947, 36.1682) -> (12.5762, 36.1682)
  arc A4533 (12.5762, 36.1682) -> (12.5762, 36.0158) centre (12.5762, 36.092) ccw
  line L4539 (12.5762, 36.0158) -> (13.6947, 36.0158)
  arc A4534 (13.6947, 36.0158) -> (13.6947, 36.1682) centre (13.6947, 36.092) ccw
  line L4540 (12.6524, 36.092) -> (12.6524, 36.8377)
  arc A4535 (12.6524, 36.8377) -> (12.5, 36.8377) centre (12.5762, 36.8377) ccw
  line L4541 (12.5, 36.8377) -> (12.5, 36.092)
  arc A4536 (12.5, 36.092) -> (12.6524, 36.092) centre (12.5762, 36.092) ccw
  line L4542 (13.6185, 37.8205) -> (13.6185, 37.4477)
  arc A4537 (13.6185, 37.4477) -> (13.7709, 37.4477) centre (13.6947, 37.4477) ccw
  arc A4538 (13.7709, 37.8205) -> (13.6185, 37.8205) centre (13.6947, 37.8205) ccw
  line L4543 (13.6408, 37.5016) -> (13.4544, 37.3152)
  arc A4539 (13.4544, 37.3152) -> (13.5622, 37.2074) centre (13.5083, 37.2613) ccw
  line L4544 (13.5622, 37.2074) -> (13.7486, 37.3938)
  arc A4540 (13.7486, 37.3938) -> (13.6408, 37.5016) centre (13.6947, 37.4477) ccw
  line L4545 (13.5083, 37.3375) -> (12.7626, 37.3375)
  arc A4541 (12.7626, 37.3375) -> (12.7626, 37.1851) centre (12.7626, 37.2613) ccw
  line L4546 (12.7626, 37.1851) -> (13.5083, 37.1851)
  arc A4542 (13.5083, 37.1851) -> (13.5083, 37.3375) centre (13.5083, 37.2613) ccw
  line L4547 (12.8165, 37.3152) -> (12.6301, 37.5016)
  arc A4543 (12.6301, 37.5016) -> (12.5223, 37.3938) centre (12.5762, 37.4477) ccw
  line L4548 (12.5223, 37.3938) -> (12.7087, 37.2074)
  arc A4544 (12.7087, 37.2074) -> (12.8165, 37.3152) centre (12.7626, 37.2613) ccw
  line L4549 (12.6524, 37.4477) -> (12.6524, 37.8205)
  arc A4545 (12.6524, 37.8205) -> (12.5, 37.8205) centre (12.5762, 37.8205) ccw
  line L4550 (12.5, 37.8205) -> (12.5, 37.4477)
  arc A4546 (12.5, 37.4477) -> (12.6524, 37.4477) centre (12.5762, 37.4477) ccw
  line L4551 (12.6301, 37.7666) -> (12.8165, 37.9531)
  arc A4547 (12.8165, 37.9531) -> (12.7087, 38.0609) centre (12.7626, 38.007) ccw
  line L4552 (12.7087, 38.0609) -> (12.5223, 37.8744)
  arc A4548 (12.5223, 37.8744) -> (12.6301, 37.7666) centre (12.5762, 37.8205) ccw
  line L4553 (12.7626, 37.9308) -> (13.5083, 37.9308)
  arc A4549 (13.5083, 37.9308) -> (13.5083, 38.0832) centre (13.5083, 38.007) ccw
  line L4554 (13.5083, 38.0832) -> (12.7626, 38.0832)
  arc A4550 (12.7626, 38.0832) -> (12.7626, 37.9308) centre (12.7626, 38.007) ccw
  line L4555 (13.4544, 37.9531) -> (13.6408, 37.7666)
  arc A4551 (13.6408, 37.7666) -> (13.7486, 37.8744) centre (13.6947, 37.8205) ccw
  line L4556 (13.7486, 37.8744) -> (13.5622, 38.0609)
  arc A4552 (13.5622, 38.0609) -> (13.4544, 37.9531) centre (13.5083, 38.007) ccw
  line L4557 (13.6185, 38.9898) -> (13.6185, 38.617)
  arc A4553 (13.6185, 38.617) -> (13.7709, 38.617) centre (13.6947, 38.617) ccw
  line L4558 (13.7709, 38.617) -> (13.7709, 38.9898)
  arc A4554 (13.7709, 38.9898) -> (13.6185, 38.9898) centre (13.6947, 38.9898) ccw
  line L4559 (13.6408, 38.6709) -> (13.4544, 38.4845)
  arc A4555 (13.4544, 38.4845) -> (13.5622, 38.3767) centre (13.5083, 38.4306) ccw
  line L4560 (13.5622, 38.3767) -> (13.7486, 38.5631)
  arc A4556 (13.7486, 38.5631) -> (13.6408, 38.6709) centre (13.6947, 38.617) ccw
  line L4561 (13.5083, 38.5068) -> (12.7626, 38.5068)
  arc A4557 (12.7626, 38.5068) -> (12.7626, 38.3544) centre (12.7626, 38.4306) ccw
  line L4562 (12.7626, 38.3544) -> (13.5083, 38.3544)
  arc A4558 (13.5083, 38.3544) -> (13.5083, 38.5068) centre (13.5083, 38.4306) ccw
  line L4563 (12.8165, 38.4845) -> (12.6301, 38.6709)
  arc A4559 (12.6301, 38.6709) -> (12.5223, 38.5631) centre (12.5762, 38.617) ccw
  line L4564 (12.5223, 38.5631) -> (12.7087, 38.3767)
  arc A4560 (12.7087, 38.3767) -> (12.8165, 38.4845) centre (12.7626, 38.4306) ccw
  line L4565 (12.6524, 38.617) -> (12.6524, 38.9898)
  arc A4561 (12.6524, 38.9898) -> (12.5, 38.9898) centre (12.5762, 38.9898) ccw
  line L4566 (12.5, 38.9898) -> (12.5, 38.617)
  arc A4562 (12.5, 38.617) -> (12.6524, 38.617) centre (12.5762, 38.617) ccw
  line L4567 (12.6301, 38.9359) -> (12.8165, 39.1224)
  arc A4563 (12.8165, 39.1224) -> (12.7087, 39.2302) centre (12.7626, 39.1763) ccw
  line L4568 (12.7087, 39.2302) -> (12.5223, 39.0437)
  arc A4564 (12.5223, 39.0437) -> (12.6301, 38.9359) centre (12.5762, 38.9898) ccw
  line L4569 (12.7626, 39.1001) -> (13.5083, 39.1001)
  arc A4565 (13.5083, 39.1001) -> (13.5083, 39.2525) centre (13.5083, 39.1763) ccw
  line L4570 (13.5083, 39.2525) -> (12.7626, 39.2525)
  arc A4566 (12.7626, 39.2525) -> (12.7626, 39.1001) centre (12.7626, 39.1763) ccw
  line L4571 (13.4544, 39.1224) -> (13.6408, 38.9359)
  arc A4567 (13.6408, 38.9359) -> (13.7486, 39.0437) centre (13.6947, 38.9898) ccw
  line L4572 (13.7486, 39.0437) -> (13.5622, 39.2302)
  arc A4568 (13.5622, 39.2302) -> (13.4544, 39.1224) centre (13.5083, 39.1763) ccw
  line L4573 (12.6185, 39.5365) -> (13.737, 40.2822)
  arc A4569 (13.737, 40.2822) -> (13.6524, 40.409) centre (13.6947, 40.3456) ccw
  line L4574 (13.6524, 40.409) -> (12.5339, 39.6633)
  arc A4570 (12.5339, 39.6633) -> (12.6185, 39.5365) centre (12.5762, 39.5999) ccw
  line L4575 (12.6524, 40.7692) -> (12.6524, 41.142)
  arc A4571 (12.6524, 41.142) -> (12.5, 41.142) centre (12.5762, 41.142) ccw
  line L4576 (12.5, 41.142) -> (12.5, 40.7692)
  arc A4572 (12.5, 40.7692) -> (12.6524, 40.7692) centre (12.5762, 40.7692) ccw
  line L4577 (12.5762, 40.8794) -> (13.6947, 40.8794)
  arc A4573 (13.6947, 40.8794) -> (13.6947, 41.0318) centre (13.6947, 40.9556) ccw
  line L4578 (13.6947, 41.0318) -> (12.5762, 41.0318)
  arc A4574 (12.5762, 41.0318) -> (12.5762, 40.8794) centre (12.5762, 40.9556) ccw
  line L4579 (13.7709, 40.7692) -> (13.7709, 41.142)
  arc A4575 (13.7709, 41.142) -> (13.6185, 41.142) centre (13.6947, 41.142) ccw
  line L4580 (13.6185, 41.142) -> (13.6185, 40.7692)
  arc A4576 (13.6185, 40.7692) -> (13.7709, 40.7692) centre (13.6947, 40.7692) ccw
  line L4581 (12.7626, 41.4725) -> (13.5083, 41.4725)
  arc A4577 (13.5083, 41.4725) -> (13.5083, 41.6249) centre (13.5083, 41.5487) ccw
  line L4582 (13.5083, 41.6249) -> (12.7626, 41.6249)
  arc A4578 (12.7626, 41.6249) -> (12.7626, 41.4725) centre (12.7626, 41.5487) ccw
  line L4583 (13.5622, 41.4948) -> (13.7486, 41.6812)
  arc A4579 (13.7486, 41.6812) -> (13.6408, 41.789) centre (13.6947, 41.7351) ccw
  line L4584 (13.6408, 41.789) -> (13.4544, 41.6026)
  arc A4580 (13.4544, 41.6026) -> (13.5622, 41.4948) centre (13.5083, 41.5487) ccw
  line L4585 (13.7709, 41.7351) -> (13.7709, 42.1079)
  arc A4581 (13.7709, 42.1079) -> (13.6185, 42.1079) centre (13.6947, 42.1079) ccw
  line L4586 (13.6185, 42.1079) -> (13.6185, 41.7351)
  arc A4582 (13.6185, 41.7351) -> (13.7709, 41.7351) centre (13.6947, 41.7351) ccw
  line L4587 (13.7486, 42.1618) -> (13.5622, 42.3483)
  arc A4583 (13.5622, 42.3483) -> (13.4544, 42.2405) centre (13.5083, 42.2944) ccw
  line L4588 (13.4544, 42.2405) -> (13.6408, 42.054)
  arc A4584 (13.6408, 42.054) -> (13.7486, 42.1618) centre (13.6947, 42.1079) ccw
  line L4589 (13.5083, 42.3706) -> (12.7626, 42.3706)
  arc A4585 (12.7626, 42.3706) -> (12.7626, 42.2182) centre (12.7626, 42.2944) ccw
  line L4590 (12.7626, 42.2182) -> (13.5083, 42.2182)
  arc A4586 (13.5083, 42.2182) -> (13.5083, 42.3706) centre (13.5083, 42.2944) ccw
  line L4591 (12.7087, 42.3483) -> (12.5223, 42.1618)
  arc A4587 (12.5223, 42.1618) -> (12.6301, 42.054) centre (12.5762, 42.1079) ccw
  line L4592 (12.6301, 42.054) -> (12.8165, 42.2405)
  arc A4588 (12.8165, 42.2405) -> (12.7087, 42.3483) centre (12.7626, 42.2944) ccw
  line L4593 (12.5, 42.1079) -> (12.5, 41.7351)
  arc A4589 (12.5, 41.7351) -> (12.6524, 41.7351) centre (12.5762, 41.7351) ccw
  line L4594 (12.6524, 41.7351) -> (12.6524, 42.1079)
  arc A4590 (12.6524, 42.1079) -> (12.5, 42.1079) centre (12.5762, 42.1079) ccw
  line L4595 (12.5223, 41.6812) -> (12.7087, 41.4948)
  arc A4591 (12.7087, 41.4948) -> (12.8165, 41.6026) centre (12.7626, 41.5487) ccw
  line L4596 (12.8165, 41.6026) -> (12.6301, 41.789)
  arc A4592 (12.6301, 41.789) -> (12.5223, 41.6812) centre (12.5762, 41.7351) ccw
  line L4597 (13.0029, 41.9754) -> (12.6301, 42.3483)
  arc A4593 (12.6301, 42.3483) -> (12.5223, 42.2405) centre (12.5762, 42.2944) ccw
  line L4598 (12.5223, 42.2405) -> (12.8951, 41.8676)
  arc A4594 (12.8951, 41.8676) -> (13.0029, 41.9754) centre (12.949, 41.9215) ccw
  line L4599 (13.4544, 43.4098) -> (13.6408, 43.2233)
  arc A4595 (13.6408, 43.2233) -> (13.7486, 43.3311) centre (13.6947, 43.2772) ccw
  line L4600 (13.7486, 43.3311) -> (13.5622, 43.5176)
  arc A4596 (13.5622, 43.5176) -> (13.4544, 43.4098) centre (13.5083, 43.4637) ccw
  line L4601 (13.6185, 43.2772) -> (13.6185, 42.9044)
  arc A4597 (13.6185, 42.9044) -> (13.7709, 42.9044) centre (13.6947, 42.9044) ccw
  line L4602 (13.7709, 42.9044) -> (13.7709, 43.2772)
  arc A4598 (13.7709, 43.2772) -> (13.6185, 43.2772) centre (13.6947, 43.2772) ccw
  line L4603 (13.6408, 42.9583) -> (13.4544, 42.7719)
  arc A4599 (13.4544, 42.7719) -> (13.5622, 42.6641) centre (13.5083, 42.718) ccw
  line L4604 (13.5622, 42.6641) -> (13.7486, 42.8505)
  arc A4600 (13.7486, 42.8505) -> (13.6408, 42.9583) centre (13.6947, 42.9044) ccw
  line L4605 (13.5083, 42.7942) -> (12.7626, 42.7942)
  arc A4601 (12.7626, 42.7942) -> (12.7626, 42.6418) centre (12.7626, 42.718) ccw
  line L4606 (12.7626, 42.6418) -> (13.5083, 42.6418)
  arc A4602 (13.5083, 42.6418) -> (13.5083, 42.7942) centre (13.5083, 42.718) ccw
  line L4607 (12.8165, 42.7719) -> (12.6301, 42.9583)
  arc A4603 (12.6301, 42.9583) -> (12.5223, 42.8505) centre (12.5762, 42.9044) ccw
  line L4608 (12.5223, 42.8505) -> (12.7087, 42.6641)
  arc A4604 (12.7087, 42.6641) -> (12.8165, 42.7719) centre (12.7626, 42.718) ccw
  line L4609 (12.6524, 42.9044) -> (12.6524, 43.2772)
  arc A4605 (12.6524, 43.2772) -> (12.5, 43.2772) centre (12.5762, 43.2772) ccw
  line L4610 (12.5, 43.2772) -> (12.5, 42.9044)
  arc A4606 (12.5, 42.9044) -> (12.6524, 42.9044) centre (12.5762, 42.9044) ccw
  line L4611 (12.6301, 43.2233) -> (12.8165, 43.4098)
  arc A4607 (12.8165, 43.4098) -> (12.7087, 43.5176) centre (12.7626, 43.4637) ccw
  line L4612 (12.7087, 43.5176) -> (12.5223, 43.3311)
  arc A4608 (12.5223, 43.3311) -> (12.6301, 43.2233) centre (12.5762, 43.2772) ccw
  line L4613 (10.5762, 28.3) -> (11.6947, 28.3)
  arc A4609 (11.6947, 28.3) -> (11.6947, 28.4524) centre (11.6947, 28.3762) ccw
  line L4614 (11.6947, 28.4524) -> (10.5762, 28.4524)
  arc A4610 (10.5762, 28.4524) -> (10.5762, 28.3) centre (10.5762, 28.3762) ccw
  line L4615 (11.7709, 28.3762) -> (11.7709, 28.9354)
  arc A4611 (11.7709, 28.9354) -> (11.6185, 28.9354) centre (11.6947, 28.9354) ccw
  line L4616 (11.6185, 28.9354) -> (11.6185, 28.3762)
  arc A4612 (11.6185, 28.3762) -> (11.7709, 28.3762) centre (11.6947, 28.3762) ccw
  line L4617 (11.7486, 28.9893) -> (11.5622, 29.1758)
  arc A4613 (11.5622, 29.1758) -> (11.4544, 29.068) centre (11.5083, 29.1219) ccw
  line L4618 (11.4544, 29.068) -> (11.6408, 28.8815)
  arc A4614 (11.6408, 28.8815) -> (11.7486, 28.9893) centre (11.6947, 28.9354) ccw
  line L4619 (11.5083, 29.1981) -> (11.1354, 29.1981)
  arc A4615 (11.1354, 29.1981) -> (11.1354, 29.0457) centre (11.1354, 29.1219) ccw
  line L4620 (11.1354, 29.0457) -> (11.5083, 29.0457)
  arc A4616 (11.5083, 29.0457) -> (11.5083, 29.1981) centre (11.5083, 29.1219) ccw
  line L4621 (11.0815, 29.1758) -> (10.8951, 28.9893)
  arc A4617 (10.8951, 28.9893) -> (11.0029, 28.8815) centre (10.949, 28.9354) ccw
  line L4622 (11.0029, 28.8815) -> (11.1893, 29.068)
  arc A4618 (11.1893, 29.068) -> (11.0815, 29.1758) centre (11.1354, 29.1219) ccw
  line L4623 (10.8728, 28.9354) -> (10.8728, 28.3762)
  arc A4619 (10.8728, 28.3762) -> (11.0252, 28.3762) centre (10.949, 28.3762) ccw
  line L4624 (11.0252, 28.3762) -> (11.0252, 28.9354)
  arc A4620 (11.0252, 28.9354) -> (10.8728, 28.9354) centre (10.949, 28.9354) ccw
  line L4625 (11.0029, 28.8029) -> (10.6301, 29.1758)
  arc A4621 (10.6301, 29.1758) -> (10.5223, 29.068) centre (10.5762, 29.1219) ccw
  line L4626 (10.5223, 29.068) -> (10.8951, 28.6951)
  arc A4622 (10.8951, 28.6951) -> (11.0029, 28.8029) centre (10.949, 28.749) ccw
  line L4627 (11.6185, 30.2912) -> (11.6185, 29.5455)
  arc A4623 (11.6185, 29.5455) -> (11.7709, 29.5455) centre (11.6947, 29.5455) ccw
  line L4628 (11.7709, 29.5455) -> (11.7709, 30.2912)
  arc A4624 (11.7709, 30.2912) -> (11.6185, 30.2912) centre (11.6947, 30.2912) ccw
  line L4629 (11.6947, 29.6217) -> (10.5762, 29.6217)
  arc A4625 (10.5762, 29.6217) -> (10.5762, 29.4693) centre (10.5762, 29.5455) ccw
  line L4630 (10.5762, 29.4693) -> (11.6947, 29.4693)
  arc A4626 (11.6947, 29.4693) -> (11.6947, 29.6217) centre (11.6947, 29.5455) ccw
  line L4631 (10.6524, 29.5455) -> (10.6524, 30.2912)
  arc A4627 (10.6524, 30.2912) -> (10.5, 30.2912) centre (10.5762, 30.2912) ccw
  line L4632 (10.5, 30.2912) -> (10.5, 29.5455)
  arc A4628 (10.5, 29.5455) -> (10.6524, 29.5455) centre (10.5762, 29.5455) ccw
  line L4633 (11.2116, 29.5455) -> (11.2116, 29.9183)
  arc A4629 (11.2116, 29.9183) -> (11.0592, 29.9183) centre (11.1354, 29.9183) ccw
  line L4634 (11.0592, 29.9183) -> (11.0592, 29.5455)
  arc A4630 (11.0592, 29.5455) -> (11.2116, 29.5455) centre (11.1354, 29.5455) ccw
  line L4635 (11.6947, 30.791) -> (10.949, 30.791)
  arc A4631 (10.949, 30.791) -> (10.949, 30.6386) centre (10.949, 30.7148) ccw
  line L4636 (10.949, 30.6386) -> (11.6947, 30.6386)
  arc A4632 (11.6947, 30.6386) -> (11.6947, 30.791) centre (11.6947, 30.7148) ccw
  line L4637 (11.0029, 30.7687) -> (10.6301, 31.1415)
  arc A4633 (10.6301, 31.1415) -> (10.5223, 31.0337) centre (10.5762, 31.0876) ccw
  line L4638 (10.5223, 31.0337) -> (10.8951, 30.6609)
  arc A4634 (10.8951, 30.6609) -> (11.0029, 30.7687) centre (10.949, 30.7148) ccw
  line L4639 (10.6301, 31.0337) -> (11.0029, 31.4066)
  arc A4635 (11.0029, 31.4066) -> (10.8951, 31.5144) centre (10.949, 31.4605) ccw
  line L4640 (10.8951, 31.5144) -> (10.5223, 31.1415)
  arc A4636 (10.5223, 31.1415) -> (10.6301, 31.0337) centre (10.5762, 31.0876) ccw
  line L4641 (10.949, 31.3843) -> (11.6947, 31.3843)
  arc A4637 (11.6947, 31.3843) -> (11.6947, 31.5367) centre (11.6947, 31.4605) ccw
  line L4642 (11.6947, 31.5367) -> (10.949, 31.5367)
  arc A4638 (10.949, 31.5367) -> (10.949, 31.3843) centre (10.949, 31.4605) ccw
  line L4643 (10.5762, 32.9772) -> (11.3219, 32.9772)
  arc A4639 (11.3219, 32.9772) -> (11.3219, 33.1296) centre (11.3219, 33.0534) ccw
  line L4644 (11.3219, 33.1296) -> (10.5762, 33.1296)
  arc A4640 (10.5762, 33.1296) -> (10.5762, 32.9772) centre (10.5762, 33.0534) ccw
  line L4645 (11.3758, 32.9995) -> (11.7486, 33.3723)
  arc A4641 (11.7486, 33.3723) -> (11.6408, 33.4801) centre (11.6947, 33.4262) ccw
  line L4646 (11.6408, 33.4801) -> (11.268, 33.1073)
  arc A4642 (11.268, 33.1073) -> (11.3758, 32.9995) centre (11.3219, 33.0534) ccw
  line L4647 (11.7486, 33.4801) -> (11.3758, 33.853)
  arc A4643 (11.3758, 33.853) -> (11.268, 33.7452) centre (11.3219, 33.7991) ccw
  line L4648 (11.268, 33.7452) -> (11.6408, 33.3723)
  arc A4644 (11.6408, 33.3723) -> (11.7486, 33.4801) centre (11.6947, 33.4262) ccw
  line L4649 (11.3219, 33.8753) -> (10.5762, 33.8753)
  arc A4645 (10.5762, 33.8753) -> (10.5762, 33.7229) centre (10.5762, 33.7991) ccw
  line L4650 (10.5762, 33.7229) -> (11.3219, 33.7229)
  arc A4646 (11.3219, 33.7229) -> (11.3219, 33.8753) centre (11.3219, 33.7991) ccw
  line L4651 (11.2116, 33.0534) -> (11.2116, 33.7991)
  arc A4647 (11.2116, 33.7991) -> (11.0592, 33.7991) centre (11.1354, 33.7991) ccw
  line L4652 (11.0592, 33.7991) -> (11.0592, 33.0534)
  arc A4648 (11.0592, 33.0534) -> (11.2116, 33.0534) centre (11.1354, 33.0534) ccw
  line L4653 (16.3922, 1.3588) -> (16.5786, 1.5452)
  arc A4649 (16.5786, 1.5452) -> (16.4708, 1.653) centre (16.5247, 1.5991) ccw
  line L4654 (16.4708, 1.653) -> (16.2844, 1.4666)
  arc A4650 (16.2844, 1.4666) -> (16.3922, 1.3588) centre (16.3383, 1.4127) ccw
  line L4655 (16.6009, 1.5991) -> (16.6009, 1.9719)
  arc A4651 (16.6009, 1.9719) -> (16.4485, 1.9719) centre (16.5247, 1.9719) ccw
  line L4656 (16.4485, 1.9719) -> (16.4485, 1.5991)
  arc A4652 (16.4485, 1.5991) -> (16.6009, 1.5991) centre (16.5247, 1.5991) ccw
  line L4657 (16.5786, 2.0258) -> (16.3922, 2.2123)
  arc A4653 (16.3922, 2.2123) -> (16.2844, 2.1045) centre (16.3383, 2.1584) ccw
  line L4658 (16.2844, 2.1045) -> (16.4708, 1.918)
  arc A4654 (16.4708, 1.918) -> (16.5786, 2.0258) centre (16.5247, 1.9719) ccw
  line L4659 (16.3383, 2.2346) -> (16.1519, 2.2346)
  line L4660 (13.7709, 37.4477) -> (13.7709, 37.8205)
  arc A4655 (16.1519, 2.2346) -> (16.1519, 2.0822) centre (16.1519, 2.1584) ccw
  line L4661 (16.1519, 2.0822) -> (16.3383, 2.0822)
  arc A4656 (16.3383, 2.0822) -> (16.3383, 2.2346) centre (16.3383, 2.1584) ccw
  line L4662 (16.098, 2.2123) -> (15.9115, 2.0258)
  arc A4657 (15.9115, 2.0258) -> (16.0193, 1.918) centre (15.9654, 1.9719) ccw
  line L4663 (16.0193, 1.918) -> (16.2058, 2.1045)
  arc A4658 (16.2058, 2.1045) -> (16.098, 2.2123) centre (16.1519, 2.1584) ccw
  line L4664 (15.8892, 1.9719) -> (15.8892, 1.7855)
  arc A4659 (15.8892, 1.7855) -> (16.0416, 1.7855) centre (15.9654, 1.7855) ccw
  line L4665 (16.0416, 1.7855) -> (16.0416, 1.9719)
  arc A4660 (16.0416, 1.9719) -> (15.8892, 1.9719) centre (15.9654, 1.9719) ccw
  line L4666 (16.0193, 2.0258) -> (15.8329, 2.2123)
  arc A4661 (13.4383, 7.9349) -> (13.4383, 8.0873) centre (13.4383, 8.0111) ccw
  arc A4662 (15.8329, 2.2123) -> (15.7251, 2.1045) centre (15.779, 2.1584) ccw
  line L4667 (15.7251, 2.1045) -> (15.9115, 1.918)
  arc A4663 (15.9115, 1.918) -> (16.0193, 2.0258) centre (15.9654, 1.9719) ccw
  line L4668 (15.779, 2.2346) -> (15.5926, 2.2346)
  arc A4664 (15.5926, 2.2346) -> (15.5926, 2.0822) centre (15.5926, 2.1584) ccw
  line L4669 (15.5926, 2.0822) -> (15.779, 2.0822)
  arc A4665 (15.779, 2.0822) -> (15.779, 2.2346) centre (15.779, 2.1584) ccw
  line L4670 (15.5387, 2.2123) -> (15.3523, 2.0258)
  arc A4666 (15.3523, 2.0258) -> (15.4601, 1.918) centre (15.4062, 1.9719) ccw
  line L4671 (15.4601, 1.918) -> (15.6465, 2.1045)
  arc A4667 (15.6465, 2.1045) -> (15.5387, 2.2123) centre (15.5926, 2.1584) ccw
  line L4672 (15.33, 1.9719) -> (15.33, 1.5991)
  arc A4668 (15.33, 1.5991) -> (15.4824, 1.5991) centre (15.4062, 1.5991) ccw
  line L4673 (15.4824, 1.5991) -> (15.4824, 1.9719)
  arc A4669 (15.4824, 1.9719) -> (15.33, 1.9719) centre (15.4062, 1.9719) ccw
  line L4674 (15.3523, 1.5452) -> (15.5387, 1.3588)
  arc A4670 (15.5387, 1.3588) -> (15.6465, 1.4666) centre (15.5926, 1.4127) ccw
  line L4675 (15.6465, 1.4666) -> (15.4601, 1.653)
  arc A4671 (15.4601, 1.653) -> (15.3523, 1.5452) centre (15.4062, 1.5991) ccw
  line L4676 (15.4062, 2.5058) -> (15.5926, 2.5058)
  arc A4672 (15.5926, 2.5058) -> (15.5926, 2.6582) centre (15.5926, 2.582) ccw
  line L4677 (15.5926, 2.6582) -> (15.4062, 2.6582)
  arc A4673 (15.4062, 2.6582) -> (15.4062, 2.5058) centre (15.4062, 2.582) ccw
  line L4678 (15.6688, 2.582) -> (15.6688, 2.7684)
  arc A4674 (15.6688, 2.7684) -> (15.5164, 2.7684) centre (15.5926, 2.7684) ccw
  line L4679 (15.5164, 2.7684) -> (15.5164, 2.582)
  arc A4675 (15.5164, 2.582) -> (15.6688, 2.582) centre (15.5926, 2.582) ccw
  line L4680 (15.5926, 2.8446) -> (15.4062, 2.8446)
  arc A4676 (15.4062, 2.8446) -> (15.4062, 2.6922) centre (15.4062, 2.7684) ccw
  line L4681 (15.4062, 2.6922) -> (15.5926, 2.6922)
  arc A4677 (15.5926, 2.6922) -> (15.5926, 2.8446) centre (15.5926, 2.7684) ccw
  line L4682 (15.33, 2.7684) -> (15.33, 2.582)
  arc A4678 (15.33, 2.582) -> (15.4824, 2.582) centre (15.4062, 2.582) ccw
  line L4683 (15.4824, 2.582) -> (15.4824, 2.7684)
  arc A4679 (15.4824, 2.7684) -> (15.33, 2.7684) centre (15.4062, 2.7684) ccw